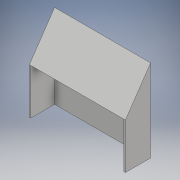
# Autodesk Inventor part: Chassi_Top_Rear
Saved by Autodesk Inventor 2018.2 (Build 222227000, 227)
## iProperties
Created: 2018-08-12
Part Number: Chassi_Top_Rear
Material: Generic
Document SubType Name: Modeling
Designer: mateu
Density: 1 g/cm^3
Appearance: Default
Author: mateu
Autodesk Inventor part; units mm, degrees
ref_plane "YZ Plane" through (0, 0, 0) normal (1, 0, 0) x (0, 1, 0)
ref_plane "XZ Plane" through (0, 0, 0) normal (0, 1, 0) x (-1, 0, 0)
ref_plane "XY Plane" through (0, 0, 0) normal (0, 0, 1) x (1, 0, 0)
sketch "Sketch1" plane through (0, 0, 0) normal (0, 0, 1) x (1, 0, 0)
  line L0 (0, 0) -> (0, -40.9)
  line L1 (0, 0) -> (156, 0)
  line L2 (156, 0) -> (156, -40.9)
  line L3 (156, -40.9) -> (153.6, -40.9)
  line L4 (153.6, -40.9) -> (153.6, -2.4)
  line L5 (153.6, -2.4) -> (2.4, -2.4)
  line L6 (2.4, -2.4) -> (2.4, -40.9)
  line L7 (2.4, -40.9) -> (0, -40.9)
  dimension "d0" = 40.9
  dimension "d1" = 156
  dimension "d2" = 2.4
  dimension "d3" = 38.5
  dimension "d4" = 151.2
  constraints: 16 end point, 4 perpendicular, 2 parallel, 1 horizontal, 1 point on line, 1 vertical
  measures "d0" distance of L0.start L0.end
  measures "d1" distance of L0.start L1.end
  measures "d2" distance of L2.end L3.end
  measures "d3" distance of L3.end L4.end
  measures "d4" distance of L4.end L5.end
extrude "Extrusion1" add sketch "Sketch1" along normal blind 73.9
sketch "Sketch2" plane through (156, -40.9, 0) normal (1, 0, 0) x (0, 0, -1)
  line L0 (-73.9, 40.9) -> (-73.9, 0) projected
  line L1 (-73.9, 40.9001) -> (-73.9, 0)
  line L2 (-73.9, 0) -> (-133.9, 40.9001)
  line L3 (-133.9, 40.9001) -> (-73.9, 40.9001)
  point P0 (0, 40.9)
  dimension "d12" = 60
  constraints: 6 end point, 1 collinear, 1 perpendicular
  measures "d12" distance of L2.end L1.start
extrude "Extrusion2" add sketch "Sketch2" against normal blind 2.4
sketch "Sketch3" plane through (0, -40.9, 0) normal (-1, 0, 0) x (0, 0, 1)
  line L0 (73.9, 38.5) -> (73.9, 40.9) projected
  line L1 (73.9, 40.9) -> (73.9, 0)
  line L2 (73.9, 0) -> (133.9, 40.9001) projected
  line L3 (73.9, 0) -> (133.9, 40.9001)
  line L4 (133.9, 40.9001) -> (73.9, 40.9)
  point P0 (0, 40.9)
  constraints: 6 end point, 1 collinear, 1 vertical
extrude "Extrusion3" add sketch "Sketch3" against normal blind 2.4
sketch "Sketch5" plane through (156, -40.9, 0) normal (1, 0, 0) x (0, 0, -1)
  line L0 (-133.9, 40.9001) -> (-73.9, 40.9001) projected
  line L1 (-73.9, 40.9001) -> (-73.9, 38.5001)
  line L2 (-73.9, 38.5) -> (-73.9, 40.9) projected
  line L3 (-73.9, 0) -> (-133.9, 40.9001) projected
  line L4 (-130.3792, 38.5001) -> (-133.9, 40.9001)
  line L5 (0, 0) -> (-73.9, 0) projected
  line L6 (-73.9, 0) -> (-73.9, 2.185)
  line L7 (-73.9, 2.185) -> (-127.1737, 38.5)
  line L8 (-127.1737, 38.5) -> (-73.9, 38.5)
  line L9 (-73.9, 0) -> (-133.9, 40.9001) projected
  point P0 (0, 40.9)
  dimension "d13" = 2.4
  constraints: 10 end point, 2 point on line, 1 collinear, 1 parallel, 1 perpendicular, 1 vertical
  measures "d13" distance of L0.end L1.end
extrude "Extrusion4" add sketch "Sketch5" against normal blind 156
body "Solid1"
